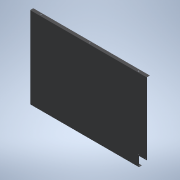
# Autodesk Inventor part: SP41V1 Cubre Base
Saved by Autodesk Inventor 2021.2 (Build 252289000, 289)
## iProperties
Created: 2026-08-25
Part Number: SP41V1 Cubre Base
Material: Generic
Document SubType Name: Sheet Metal
Designer: nelso
Density: 1 g/cm^3
Sheet Metal Rule: Default_mm
Appearance: Gray
Flat Pattern Width: 57.2593 cm
Flat Pattern Length: 76.3 cm
Flat Pattern Area: 4368.89 cm^2
Sheet Metal Width: 572.593 mm
Sheet Metal Length: 763.000 mm
Sheet Metal Area: 436888.559 mm^2
Author: nelso
Autodesk Inventor part; units mm, degrees
ref_plane "YZ Plane" through (0, 0, 0) normal (1, 0, 0) x (0, 1, 0)
ref_plane "XZ Plane" through (0, 0, 0) normal (0, 1, 0) x (-1, 0, 0)
ref_plane "XY Plane" through (0, 0, 0) normal (0, 0, 1) x (1, 0, 0)
sketch "Sketch1" plane through (0, 0, 0) normal (0, 1, 0) x (-1, 0, 0)
  line L0 (381.5, 268.3) -> (-381.5, 268.3)
  line L1 (-381.5, 268.3) -> (-381.5, -268.3)
  line L2 (-381.5, -268.3) -> (381.5, -268.3)
  line L3 (381.5, -268.3) -> (381.5, 268.3)
  line L4 (381.5, 268.3) -> (-381.5, -268.3) construction
  line L5 (-381.5, 268.3) -> (381.5, -268.3) construction
  point P0 (0, 0)
  dimension "d0" = 763
  dimension "d1" = 536.6
  measures "d0" distance of L2.end L1.end
  measures "d1" distance of L1.end L0.end
extrude "Plate1" add sketch "Sketch1" along normal blind 0.9
sketch "Sketch2" plane through (381.5, 0, 267.4) normal (0, 0, 1) x (1, 0, 0)
  line L0 (-763, 0) -> (0, 0)
  line L1 (0, 0) -> (0, 20)
  line L2 (0, 20) -> (-763, 20)
  line L3 (-763, 20) -> (-763, 0)
  constraints: 6 end point, 1 horizontal, 1 perpendicular, 1 vertical
edge flange "Flange1" height 20 angle 90 thickness 0.9 bend radius 1.008 thickness toward (0, 0, 1) relief straight relief width 0.9 relief depth 0.45 corner gap 1.008 corner form 0 edges at (0, 0.9, 268.3) (0, 0.9, -268.3) wall of the first edge with corners at (-381.5, 0, 267.4) (381.5, 0, 267.4) (381.5, 20, 267.4) (-381.5, 20, 267.4)
bend "Bend1"
corner "Corner1"
sketch "Sketch3" plane through (-381.5, 20, 268.3) normal (0, 0, 1) x (1, 0, 0)
  circle A0 centre (381.5, -11) radius 1.7
  circle A1 centre (61.5, -11) radius 1.7
  line L0 (0, 0) -> (763, 0) projected
  point P0 (381.5, -20)
  point P1 (701.5, -11)
  dimension "d20" = 11
  dimension "d41" = 320
  dimension "d42" = 320
  constraints: 2 centre point, 2 coincident, 2 other
  measures "d20" distance from line of L0 point (61.5, -11)
  measures "d41" distance of point (701.5, -11) point (381.5, -11)
  measures "d42" distance of point (381.5, -11) point (61.5, -11)
hole "Hole1" at (-320, 9, 268.3) at (0, 9, 268.3) at (320, 9, 268.3) direction (0, 0, -1) diameter 6 end through all
sketch "Sketch6" plane through (0, 0, 0) normal (0, -1, 0) x (1, 0, 0)
  line L0 (381.5, -268.3) -> (-381.5, -268.3) projected
  line L1 (329.5, -203.3) -> (329.5, -268.3)
  line L2 (329.5, -268.3) -> (381.5, -268.3)
  line L3 (381.5, -268.3) -> (381.5, -203.3)
  line L4 (329.5, -203.3) -> (381.5, -203.3)
  point P0 (0, 0)
  dimension "d39" = 52
  dimension "d44" = 65
  constraints: 8 end point, 1 horizontal, 1 parallel, 1 point on line
  measures "d39" distance between parallel lines of L1 L3
  measures "d44" distance of L0.start L3.end
extrude "Cut1" cut sketch "Sketch6" against normal through all
fillet "Corner Round1" radius 2 6 edges at (329.5, 20, -267.85) (381.5, 20, 267.85) (-381.5, 20, -267.85) (-381.5, 20, 267.85) (329.5, 0.45, -203.3) (381.5, 0.45, -203.3)
sketch "Sketch8" plane through (0, 0, 0) normal (0, -1, 0) x (1, 0, 0)
  circle A0 centre (325.5, -199.3) radius 1.8 projected
  circle A1 centre (374, -197.8) radius 1.8 projected
  circle A2 centre (324, -260.5) radius 1.8 projected
  arc A3 (377, -268) -> (381.5, -263.5) centre (377, -263.5) ccw projected
  line L0 (381.5, -263.5) -> (381.5, -193.3) projected
  arc A4 (381.5, -193.3) -> (378.5, -190.3) centre (378.5, -193.3) ccw projected
  line L1 (378.5, -190.3) -> (322.5, -190.3) projected
  arc A5 (322.5, -190.3) -> (316.5, -196.3) centre (322.5, -196.3) ccw projected
  line L2 (316.5, -196.3) -> (316.5, -265) projected
  arc A6 (316.5, -265) -> (319.5, -268) centre (319.5, -265) ccw projected
  line L3 (319.5, -268) -> (377, -268) projected
  line L4 (379.5, -208.3) -> (379.5, -263) projected
  arc A7 (376.5, -266) -> (379.5, -263) centre (376.5, -263) ccw projected
  line L5 (376.5, -266) -> (334.5, -266) projected
  arc A8 (331.5, -263) -> (334.5, -266) centre (334.5, -263) ccw projected
  line L6 (331.5, -263) -> (331.5, -208.3) projected
  arc A9 (334.5, -205.3) -> (331.5, -208.3) centre (334.5, -208.3) ccw projected
  line L7 (334.5, -205.3) -> (376.5, -205.3) projected
  arc A10 (379.5, -208.3) -> (376.5, -205.3) centre (376.5, -208.3) ccw projected
  point P0 (0, 0)
  dimension "d13" = 6
  dimension "d15" = 6.3
  dimension "d16" = 2
  dimension "d18" = 0.9
  constraints: 3 coincident
hole "Hole2" at (374, 0, -197.8) at (325.5, 0, -199.3) at (324, 0, -260.5) direction (0, 1, 0) diameter 3.4 depth 0.9 tip angle 118 clearance for "Countersunk Flat Head Screw ISO 2009/7046" size "M3" standard "ISO"
equation "\"d18\" = Thickness"
equation "\"d50\" = Thickness"
equation "\"d2\" = Thickness"
equation "\"d3\" = BendReliefWidth"
equation "\"d4\" = BendReliefDepth"
equation "\"d5\" = MinimumRemnant"
equation "\"d6\" = TransitionRadius"
equation "\"d9\" = BendRadius"
equation "\"d10\" = CornerReliefSize"
equation "\"d11\" = GapSize"
equation "\"d12\" = JacobiRadiusSize"
equation "\"BendReliefWidth\" = Thickness"
equation "\"BendReliefDepth\" = 0.5 * Thickness"
equation "\"CornerReliefSize\" = 4 * Thickness"
equation "\"MinimumRemnant\" = 2 * Thickness"
equation "\"TransitionRadius\" = BendRadius"
equation "\"JacobiRadiusSize\" = BendRadius"
equation "\"GapSize\" = Thickness"
equation "\"Thickness\" = 0.9"
equation "\"BendRadius\" = 1.008"
body "Solid1"
